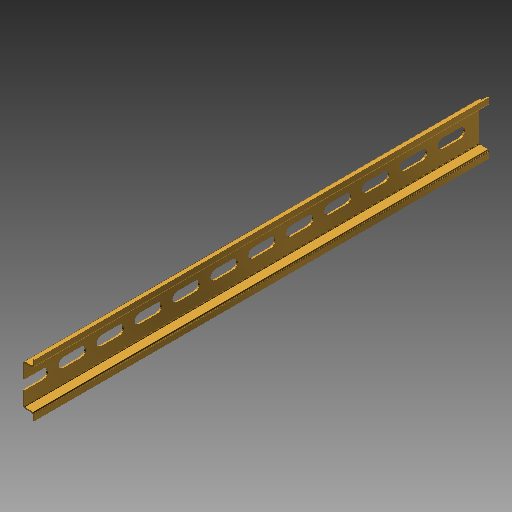
# Autodesk Inventor part: Din Rail_300
Saved by Autodesk Inventor 2019.3 (Build 233278000, 278)
## iProperties
Shininess: 64.0
Length Units: 11272
Angle Units: 11279
Time Units: 11290
Mass Units: 11286
Length Display Precision: 3
Angle Display Precision: 2
Compacted: True
Part Number: Din Rail_300
Document SubType Name: Modeling
Created: 2004-01-04
Designer: vporto
Material: Латунь светло-желтая
Manufacturer: Standard
Standards Organization: Custom
Project: PRJ0130
Description: BM AC POWER ENC DIN RAIL 3"
Mass: 25.1377 g
Surface Area: 62.1386 cm^2
Volume: 2.96785 cm^3
Density: 8.47 g/cm^3
Appearance: Латунь — сатинированная
Density: 0.0
Volumn: 0.0
Area: 0.0
PropertySet Name: Model Information
Control State: 0
Master: False
Checked Out: False
Author: JFARIA
Revision Number: A
Autodesk Inventor part; units mm, degrees
ref_plane "YZ Plane" through (0, 0, 0) normal (1, 0, 0) x (0, 1, 0)
ref_plane "XZ Plane" through (0, 0, 0) normal (0, 1, 0) x (-1, 0, 0)
ref_plane "XY Plane" through (0, 0, 0) normal (0, 0, 1) x (1, 0, 0)
sketch "Sketch2" plane through (0, 0, 0) normal (0, 0, 1) x (1, 0, 0)
  line L0 (3.5814, 15.9041) -> (4.5814, 15.9041)
  line L1 (4.5814, 15.9041) -> (4.5814, 10.9041)
  line L2 (4.5814, 10.9041) -> (-1.9186, 10.9041)
  line L3 (-1.9186, 10.9041) -> (-1.9186, -14.0959)
  line L4 (-1.9186, -14.0959) -> (4.5814, -14.0959)
  line L5 (4.5814, -14.0959) -> (4.5814, -19.0959)
  line L6 (4.5814, -19.0959) -> (3.5814, -19.0959)
  line L7 (3.5814, -19.0959) -> (3.5814, -15.0959)
  line L8 (3.5814, -15.0959) -> (-2.9186, -15.0959)
  line L9 (-2.9186, -15.0959) -> (-2.9186, 11.9041)
  line L10 (-2.9186, 11.9041) -> (3.5814, 11.9041)
  line L11 (3.5814, 11.9041) -> (3.5814, 15.9041)
  dimension "d0" = 1
  dimension "d1" = 35
  dimension "d2" = 27
  dimension "d3" = 1
  dimension "d4" = 1
  dimension "d5" = 1
  dimension "d6" = 1
  dimension "d7" = 4
  dimension "d8" = 7.5
  constraints: 24 end point, 6 parallel, 4 perpendicular, 1 collinear, 1 horizontal
  measures "d0" distance of L0.start L0.end
  measures "d1" distance between parallel lines of L6 L0
  measures "d2" distance of L8.end L9.end
  measures "d3" distance between parallel lines of L2 L10
  measures "d4" distance between parallel lines of L3 L9
  measures "d5" distance between parallel lines of L4 L8
  measures "d6" distance of L5.end L6.end
  measures "d7" distance of L10.end L0.start
  measures "d8" distance between parallel lines of L9 L1
extrude "Main" add sketch "Sketch2" along normal blind 300
fillet "Fillet2" radius 1.5875 4 edges at (4.5814, 10.9041, 150) (-2.9186, 11.9041, 150) (4.5814, -14.0959, 150) (-2.9186, -15.0959, 150)
fillet "Fillet3" radius 0.7937 4 edges at (3.5814, -15.0959, 150) (-1.9186, 10.9041, 150) (3.5814, 11.9041, 150) (-1.9186, -14.0959, 150)
sketch "Sketch3" plane through (-1.9186, -13.3022, 0) normal (1, 0, 0) x (0, 0, -1)
  line L0 (0, 23.4125) -> (0, 0) projected
  line L1 (-12.5, 8.5563) -> (-24.2, 8.5563)
  line L2 (-27.35, 11.7063) -> (-27.35, 11.7062)
  line L3 (-24.2, 14.8562) -> (-12.5, 14.8563)
  line L4 (-9.35, 11.7063) -> (-9.35, 11.7063)
  arc A0 (-24.2, 14.8562) -> (-27.35, 11.7062) centre (-24.2, 11.7062) ccw
  arc A1 (-27.35, 11.7063) -> (-24.2, 8.5563) centre (-24.2, 11.7063) ccw
  arc A2 (-12.5, 8.5563) -> (-9.35, 11.7063) centre (-12.5, 11.7063) ccw
  arc A3 (-9.35, 11.7063) -> (-12.5, 14.8563) centre (-12.5, 11.7063) ccw
  line L5 (0, 29.2063) -> (-300, 29.2063) projected
  dimension "d14" = 3.15
  dimension "d15" = 6.3
  dimension "d16" = 18
  dimension "d17" = 17.5
  dimension "d18" = 12.5
  constraints: 8 end point, 8 point on circle, 8 tangent, 4 centre point, 3 equal radius, 2 parallel, 1 horizontal, 1 perpendicular
  measures "d14" radius of A0
  measures "d15" distance between parallel lines of L3 L1
  measures "d16" distance of L4.end L2.end
  measures "d17" distance from line of A2.centre L5
  measures "d18" distance from line of A3.centre L0
extrude "Extrusion2" cut sketch "Sketch3" against normal through all
pattern_linear "Rectangular Pattern1" count 30 spacing 25 along (0, 0, 1) of "Extrusion2"
equation "\"d0\" = DINWidth"
equation "\"d1\" = DINHeight"
equation "\"d2\" = DINHeightBack"
equation "\"d3\" = DINWidth"
equation "\"d4\" = DINWidth"
equation "\"d5\" = DINWidth"
equation "\"d6\" = DINWidth"
equation "\"d7\" = -0.5 * d2 + 0.5 * d1"
equation "\"d8\" = DINDepth"
equation "\"d14\" = 0.5 * SlotHeight"
equation "\"d15\" = SlotHeight"
equation "\"d16\" = SlotLength"
equation "\"d17\" = 0.5 * DINHeight"
equation "\"d18\" = 0.5 * SlotSpacing"
equation "\"d23\" = SlotSpacing"
equation "\"DINLength\" = 76.2"
equation "\"DINHeight\" = 35"
equation "\"DINHeightBack\" = 27"
equation "\"DINDepth\" = 7.5"
equation "\"SlotHeight\" = 6.3"
equation "\"SlotLength\" = 18"
equation "\"SlotSpacing\" = 25"
equation "\"DINWidth\" = 1"
body "Solid1"
